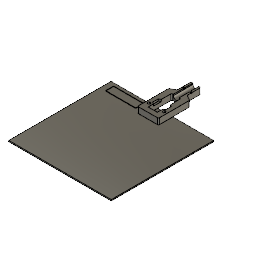
bed-strain-relief (Autodesk Fusion 360 design; units mm, degrees)
Autodesk Fusion 360 part; units mm, degrees
sketch "Sketch1" plane through (0, 0, 0) normal (0, 0, 1) x (1, 0, 0) in component "BedPlate"
  line L0 (0, 0) -> (260.35, 0)
  line L1 (260.35, 0) -> (260.35, 260.35)
  line L2 (260.35, 260.35) -> (0, 260.35)
  line L3 (0, 260.35) -> (0, 0)
  dimension "d1" = 260.35
  dimension "d2" = 260.35
  measures "d1" distance of L1 L3
  measures "d2" distance of L0 L2
extrude "Extrude1" add sketch "Sketch1" against normal blind 3.175 makes body 1 in component "BedPlate"
sketch "Sketch2" plane through (0, 0, 0) normal (0, 0, 1) x (-1, 0, 0) in component "BedPlate"
  circle A0 centre (-111.0875, -245.35) radius 1.5875
  circle A1 centre (-149.2625, -245.35) radius 1.5875
  line L0 (-118.675, -245.35) -> (-141.675, -245.35) construction
  line L1 (-260.35, -260.35) -> (0, -260.35)
  line L2 (-130.175, -260.35) -> (-130.175, -245.35) construction
  line L3 (-112.675, -245.35) -> (-147.675, -245.35)
  line L4 (-118.675, -245.35) -> (-118.675, -260.35) construction
  line L5 (-141.675, -245.35) -> (-141.675, -260.35) construction
  dimension "d5" = 23
  dimension "d7" = 3.175
  dimension "d8" = 3.175
  dimension "d9" = 6
  dimension "d10" = 15
  measures "d7" diameter of A0
  measures "d8" diameter of A1
  measures "d10" distance of L1 L3
extrude "Extrude2" cut sketch "Sketch2" against normal through all bodies 1 in component "BedPlate"
sketch "Sketch1 (2)" plane through (0, 0, 0) normal (0, 0, 1) x (-1, 0, 0) in component "WireSupportBracket"
  line L0 (-103.675, -302.2671) -> (-103.675, -223.35)
  line L1 (-103.675, -223.35) -> (-156.675, -223.35)
  line L2 (-156.675, -223.35) -> (-156.675, -302.2671)
  line L3 (-141.675, -295.35) -> (-141.675, -235.35)
  line L4 (-141.675, -235.35) -> (-118.675, -235.35)
  line L5 (-118.675, -235.35) -> (-118.675, -295.35)
  circle A0 centre (-149.2625, -245.35) radius 1.5875
  circle A1 centre (-111.0875, -245.35) radius 1.5875
  line L6 (-149.2625, -245.35) -> (-111.0875, -245.35) construction
  line L7 (-130.175, -356.4968) -> (-130.175, -223.35) construction
  line L8 (-260.35, -260.35) -> (0, -260.35) construction
  line L9 (-118.675, -295.35) -> (-141.675, -295.35)
  line L10 (-122.675, -345.35) -> (-122.675, -295.35)
  line L11 (-137.675, -295.35) -> (-137.675, -345.35)
  line L12 (-117.675, -310.35) -> (-103.675, -302.2671)
  line L13 (-156.675, -302.2671) -> (-142.675, -310.35)
  line L14 (-117.675, -310.35) -> (-117.675, -345.35)
  line L15 (-142.675, -310.35) -> (-142.675, -345.35)
  line L16 (-122.675, -313.5082) -> (-137.675, -313.5082) construction
  line L17 (-117.675, -345.35) -> (-142.675, -345.35)
  line L18 (-145.9139, -245.35) -> (-147.5882, -242.45)
  line L19 (-147.5882, -242.45) -> (-150.9368, -242.45)
  line L20 (-150.9368, -242.45) -> (-152.6111, -245.35)
  line L21 (-152.6111, -245.35) -> (-150.9368, -248.25)
  line L22 (-150.9368, -248.25) -> (-147.5882, -248.25)
  line L23 (-147.5882, -248.25) -> (-145.9139, -245.35)
  line L24 (-114.4361, -245.35) -> (-112.7618, -242.45)
  line L25 (-112.7618, -242.45) -> (-109.4132, -242.45)
  line L26 (-109.4132, -242.45) -> (-107.7389, -245.35)
  line L27 (-107.7389, -245.35) -> (-109.4132, -248.25)
  line L28 (-109.4132, -248.25) -> (-112.7618, -248.25)
  line L29 (-112.7618, -248.25) -> (-114.4361, -245.35)
  point P0 (0, 0.0158)
  dimension "d12" = 23
  dimension "d14" = 25
  dimension "d15" = 12
  dimension "d16" = 15
  dimension "d18" = 15
  dimension "d19" = 50
  dimension "d20" = 15
  dimension "d21" = 60
  dimension "d22" = 15
  dimension "d23" = 5
  dimension "d25" = 50
  dimension "d26" = 5.8
  measures "d14" distance of L4 L8
  measures "d15" distance of L1 L4
  measures "d25" distance of L9 L17
  measures "d26" distance of L19 L22
extrude "Extrude1'" add sketch "Sketch1 (2)" along normal blind 15 separate body contours L0 L1 L2 L3 L4 L5 L9 L10 L11 L12 L13 L14 L15 L17 | L9 L10 L11 L17 | L18 L19 L20 L21 L22 L23 | L24 L25 L26 L27 L28 L29 makes body 2 in component "WireSupportBracket"
extrude "Extrude2'" cut sketch "Sketch1 (2)" against normal blind 6 from surface at 15 contours L18 L19 L20 L21 L22 L23 | L24 L25 L26 L27 L28 L29 bodies 2 in component "WireSupportBracket"
sketch "Sketch2 (2)" plane through (0, 345.35, 0) normal (0, 1, 0) x (-1, 0, 0) in component "WireSupportBracket"
  circle A0 centre (-130.175, 12) radius 7.5
  line L0 (-122.675, 0) -> (-122.675, 19.5)
  line L1 (-137.675, 0) -> (-137.675, 19.5)
  line L2 (-137.675, 19.5) -> (-122.675, 19.5)
  line L3 (-117.675, 0) -> (-142.675, 0) construction
  dimension "d32" = 12
extrude "Extrude3" cut sketch "Sketch2 (2)" against normal up to surface (50 mm away) bodies 2 in component "WireSupportBracket"
ref_plane "WorkPlane1" through (130.175, 321.35, 7.5) normal (0, 1, 0) x (-1, 0, 0) in component "WireSupportBracket"
sketch "Sketch3" plane through (130.175, 321.35, 7.5) normal (0, 1, 0) x (1, 0, 0) in component "WireSupportBracket"
  arc A0 (7.5, -4.5) -> (-7.5, -4.5) centre (0, -4.5) ccw
  line L0 (7.5, -4.5) -> (7.5, -7.5)
  line L1 (-7.5, -4.5) -> (-7.5, -7.5)
  line L2 (-9.5, -4.5) -> (-9.5, -7.5)
  arc A1 (9.5, -4.5) -> (-9.5, -4.5) centre (0, -4.5) ccw
  line L3 (9.5, -4.5) -> (9.5, -7.5)
  line L4 (11, -4.5) -> (11, -7.5)
  arc A2 (11, -4.5) -> (-11, -4.5) centre (0, -4.5) ccw
  line L5 (-11, -4.5) -> (-11, -7.5)
  line L6 (-9.5, -7.5) -> (-11, -7.5)
  line L7 (11, -7.5) -> (9.5, -7.5)
  line L8 (11.5, -7.5) -> (-11.5, -7.5)
  dimension "d36" = 2
  dimension "d38" = 3.5
  measures "d36" distance of L1
  measures "d38" distance of L1 L5
extrude "Extrude4" cut sketch "Sketch3" along normal blind 3 contours L2 A1 L3 L4 A2 L5 L6 L7 L8 bodies 2 in component "WireSupportBracket"
fillet "Fillet1" radius 2.5 10 edges at (156.675, 223.35, 7.5) (156.675, 302.2671, 7.5) (142.675, 310.35, 7.5) (142.675, 345.35, 7.5) (117.675, 345.35, 7.5) (117.675, 310.35, 7.5) (103.675, 302.2671, 7.5) (103.675, 223.35, 7.5) (141.675, 295.35, 7.5) (118.675, 295.35, 7.5) on bodies 2 in component "WireSupportBracket"
sketch "Sketch3 (2)" plane through (0, 0, 0) normal (0, 0, 1) x (-1, 0, 0) in component "BedPlate"
  line L0 (-15, -251.35) -> (-91.2, -251.35)
  line L1 (-91.2, -251.35) -> (-91.2, -231.35)
  line L2 (-91.2, -231.35) -> (-15, -231.35)
  line L3 (-15, -231.35) -> (-15, -251.35)
  line L4 (0, -260.35) -> (0, 0)
  line L5 (-260.35, -260.35) -> (0, -260.35)
  dimension "d42" = 76.2
  dimension "d43" = 20
  dimension "d44" = 15
  dimension "d45" = 9
  measures "d42" distance of L4.end
  measures "d44" distance of L3 L4
  measures "d45" distance of L0 L5
extrude "Extrude3'" add sketch "Sketch3 (2)" along normal blind 1 bodies 1 in component "BedPlate"
sketch "Sketch4" plane through (0, 0, 15) normal (0, 0, 1) x (-1, 0, 0) in component "WireSupportBracket"
  line L0 (-141.675, -268.85) -> (-146.675, -265.9632)
  line L1 (-146.675, -265.9632) -> (-146.675, -251.7368)
  line L2 (-146.675, -251.7368) -> (-141.675, -248.85)
  line L3 (-106.175, -223.35) -> (-154.175, -223.35)
  line L4 (-141.675, -292.85) -> (-141.675, -235.35)
  line L5 (-130.175, -223.35) -> (-130.175, -293.582) construction
  line L6 (-146.675, -258.85) -> (-141.675, -258.85) construction
  line L7 (-118.675, -268.85) -> (-113.675, -265.9632)
  line L8 (-113.675, -265.9632) -> (-113.675, -251.7368)
  line L9 (-113.675, -251.7368) -> (-118.675, -248.85)
  line L10 (-118.675, -235.35) -> (-118.675, -292.85)
  line L11 (-141.175, -321.35) -> (-139.675, -321.35)
  line L12 (-139.675, -324.35) -> (-141.175, -324.35)
  line L13 (-137.675, -345.35) -> (-137.675, -295.35)
  line L14 (-139.675, -321.35) -> (-137.675, -320.1953)
  line L15 (-139.675, -324.35) -> (-137.675, -325.5047)
  line L16 (-137.675, -322.85) -> (-139.675, -322.85) construction
  line L17 (-139.675, -321.35) -> (-139.675, -324.35)
  line L18 (-120.675, -321.35) -> (-122.675, -320.1953)
  line L19 (-120.675, -324.35) -> (-122.675, -325.5047)
  line L20 (-120.675, -321.35) -> (-120.675, -324.35)
  line L21 (-122.675, -295.35) -> (-122.675, -345.35)
  dimension "d48" = 24
  dimension "d49" = 5
  dimension "d50" = 20
  dimension "d51" = 60
  dimension "d52" = 60
  measures "d49" distance of L1 L4
  measures "d51" angle of L2 L4
extrude "Extrude5" cut sketch "Sketch4" against normal blind 3 contours L13 L14 L15 L17 | L18 L19 L20 L21 bodies 2 in component "WireSupportBracket"
extrude "Extrude6" cut sketch "Sketch4" against normal blind 5 contours L0 L1 L2 L4 | L7 L8 L9 L10 bodies 2 in component "WireSupportBracket"
component "BedPlate" placed x (1, 0, 0) y (0, 1, 0) z (0, 0, 1) at (0, 0, 0)
component "WireSupportBracket" placed x (1, 0, 0) y (0, 1, 0) z (0, 0, 1) at (0, 0, 0)
equation "d8 = d7"
